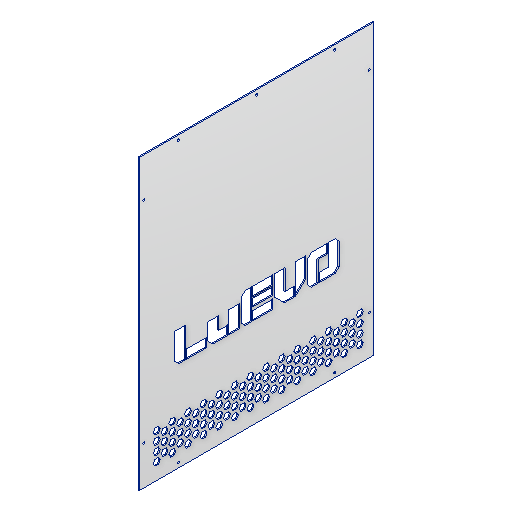
# Autodesk Inventor part: Camera Side Panel
Saved by Autodesk Inventor 2023.2 (Build 272271000, 271)
## iProperties
Created: 2023-02-06
Part Number: Camera Side Panel
Material: Aluminum 6061
Document SubType Name: Modeling
Designer: remop
Density: 2.7 g/cm^3
Appearance: Aluminum - Flat
Author: remop
Autodesk Inventor part; units mm, degrees
(part 1 of 2)
ref_plane "YZ Plane" through (0, 0, 0) normal (1, 0, 0) x (0, 1, 0)
ref_plane "XZ Plane" through (0, 0, 0) normal (0, 1, 0) x (-1, 0, 0)
ref_plane "XY Plane" through (0, 0, 0) normal (0, 0, 1) x (1, 0, 0)
sketch "Sketch1" plane through (0, 0, 0) normal (1, 0, 0) x (0, 1, 0)
  line L0 (168.0981, 15.8482) -> (163.0981, 18.735) projected
  line L1 (163.0981, 18.735) -> (163.0981, 24.5085) projected
  line L2 (163.0981, 24.5085) -> (168.0981, 27.3952) projected
  line L3 (168.0981, 27.3952) -> (173.0981, 24.5085) projected
  line L4 (173.0981, 24.5085) -> (173.0981, 18.735) projected
  line L5 (173.0981, 18.735) -> (168.0981, 15.8482) projected
  line L6 (130.5981, 40.3856) -> (135.5981, 37.4988) projected
  line L7 (135.5981, 37.4988) -> (135.5981, 31.7253) projected
  line L8 (135.5981, 31.7253) -> (130.5981, 28.8386) projected
  line L9 (130.5981, 28.8386) -> (125.5981, 31.7253) projected
  line L10 (125.5981, 31.7253) -> (125.5981, 37.4988) projected
  line L11 (125.5981, 37.4988) -> (130.5981, 40.3856) projected
  line L12 (158.0981, 50.5085) -> (158.0981, 44.735) projected
  line L13 (158.0981, 44.735) -> (153.0981, 41.8482) projected
  line L14 (153.0981, 41.8482) -> (148.0981, 44.735) projected
  line L15 (148.0981, 44.735) -> (148.0981, 50.5085) projected
  line L16 (148.0981, 50.5085) -> (153.0981, 53.3952) projected
  line L17 (153.0981, 53.3952) -> (158.0981, 50.5085) projected
  line L18 (140.5981, 63.4988) -> (145.5981, 66.3856) projected
  line L19 (145.5981, 66.3856) -> (150.5981, 63.4988) projected
  line L20 (150.5981, 63.4988) -> (150.5981, 57.7253) projected
  line L21 (150.5981, 57.7253) -> (145.5981, 54.8386) projected
  line L22 (145.5981, 54.8386) -> (140.5981, 57.7253) projected
  line L23 (140.5981, 57.7253) -> (140.5981, 63.4988) projected
  line L24 (143.0981, 70.735) -> (138.0981, 67.8482) projected
  line L25 (138.0981, 67.8482) -> (133.0981, 70.735) projected
  line L26 (133.0981, 70.735) -> (133.0981, 76.5085) projected
  line L27 (133.0981, 76.5085) -> (138.0981, 79.3952) projected
  line L28 (138.0981, 79.3952) -> (143.0981, 76.5085) projected
  line L29 (143.0981, 76.5085) -> (143.0981, 70.735) projected
  line L30 (160.5981, 92.3856) -> (165.5981, 89.4988) projected
  line L31 (165.5981, 89.4988) -> (165.5981, 83.7253) projected
  line L32 (165.5981, 83.7253) -> (160.5981, 80.8386) projected
  line L33 (160.5981, 80.8386) -> (155.5981, 83.7253) projected
  line L34 (155.5981, 83.7253) -> (155.5981, 89.4988) projected
  line L35 (155.5981, 89.4988) -> (160.5981, 92.3856) projected
  line L36 (128.0981, 102.5085) -> (128.0981, 96.735) projected
  line L37 (128.0981, 96.735) -> (123.0981, 93.8482) projected
  line L38 (123.0981, 93.8482) -> (118.0981, 96.735) projected
  line L39 (118.0981, 96.735) -> (118.0981, 102.5085) projected
  line L40 (118.0981, 102.5085) -> (123.0981, 105.3952) projected
  line L41 (123.0981, 105.3952) -> (128.0981, 102.5085) projected
  line L42 (168.0981, 119.8482) -> (163.0981, 122.735) projected
  line L43 (163.0981, 122.735) -> (163.0981, 128.5085) projected
  line L44 (163.0981, 128.5085) -> (168.0981, 131.3952) projected
  line L45 (168.0981, 131.3952) -> (173.0981, 128.5085) projected
  line L46 (173.0981, 128.5085) -> (173.0981, 122.735) projected
  line L47 (173.0981, 122.735) -> (168.0981, 119.8482) projected
  line L48 (130.5981, 144.3856) -> (135.5981, 141.4988) projected
  line L49 (135.5981, 141.4988) -> (135.5981, 135.7253) projected
  line L50 (135.5981, 135.7253) -> (130.5981, 132.8386) projected
  line L51 (130.5981, 132.8386) -> (125.5981, 135.7253) projected
  line L52 (125.5981, 135.7253) -> (125.5981, 141.4988) projected
  line L53 (125.5981, 141.4988) -> (130.5981, 144.3856) projected
  line L54 (160.5981, 144.3856) -> (165.5981, 141.4988) projected
  line L55 (165.5981, 141.4988) -> (165.5981, 135.7253) projected
  line L56 (165.5981, 135.7253) -> (160.5981, 132.8386) projected
  line L57 (160.5981, 132.8386) -> (155.5981, 135.7253) projected
  line L58 (155.5981, 135.7253) -> (155.5981, 141.4988) projected
  line L59 (155.5981, 141.4988) -> (160.5981, 144.3856) projected
  line L60 (140.5981, 167.4988) -> (145.5981, 170.3856) projected
  line L61 (145.5981, 170.3856) -> (150.5981, 167.4988) projected
  line L62 (150.5981, 167.4988) -> (150.5981, 161.7253) projected
  line L63 (150.5981, 161.7253) -> (145.5981, 158.8386) projected
  line L64 (145.5981, 158.8386) -> (140.5981, 161.7253) projected
  line L65 (140.5981, 161.7253) -> (140.5981, 167.4988) projected
  line L66 (143.0981, 174.735) -> (138.0981, 171.8482) projected
  line L67 (138.0981, 171.8482) -> (133.0981, 174.735) projected
  line L68 (133.0981, 174.735) -> (133.0981, 180.5085) projected
  line L69 (133.0981, 180.5085) -> (138.0981, 183.3952) projected
  line L70 (138.0981, 183.3952) -> (143.0981, 180.5085) projected
  line L71 (143.0981, 180.5085) -> (143.0981, 174.735) projected
  line L72 (160.5981, 196.3856) -> (165.5981, 193.4988) projected
  line L73 (165.5981, 193.4988) -> (165.5981, 187.7253) projected
  line L74 (165.5981, 187.7253) -> (160.5981, 184.8386) projected
  line L75 (160.5981, 184.8386) -> (155.5981, 187.7253) projected
  line L76 (155.5981, 187.7253) -> (155.5981, 193.4988) projected
  line L77 (155.5981, 193.4988) -> (160.5981, 196.3856) projected
  line L78 (128.0981, 206.5085) -> (128.0981, 200.735) projected
  line L79 (128.0981, 200.735) -> (123.0981, 197.8482) projected
  line L80 (123.0981, 197.8482) -> (118.0981, 200.735) projected
  line L81 (118.0981, 200.735) -> (118.0981, 206.5085) projected
  line L82 (118.0981, 206.5085) -> (123.0981, 209.3952) projected
  line L83 (123.0981, 209.3952) -> (128.0981, 206.5085) projected
  line L84 (168.0981, 223.8482) -> (163.0981, 226.735) projected
  line L85 (163.0981, 226.735) -> (163.0981, 232.5085) projected
  line L86 (163.0981, 232.5085) -> (168.0981, 235.3952) projected
  line L87 (168.0981, 235.3952) -> (173.0981, 232.5085) projected
  line L88 (173.0981, 232.5085) -> (173.0981, 226.735) projected
  line L89 (173.0981, 226.735) -> (168.0981, 223.8482) projected
  line L90 (130.5981, 248.3856) -> (135.5981, 245.4988) projected
  line L91 (135.5981, 245.4988) -> (135.5981, 239.7253) projected
  line L92 (135.5981, 239.7253) -> (130.5981, 236.8386) projected
  line L93 (130.5981, 236.8386) -> (125.5981, 239.7253) projected
  line L94 (125.5981, 239.7253) -> (125.5981, 245.4988) projected
  line L95 (125.5981, 245.4988) -> (130.5981, 248.3856) projected
  line L96 (158.0981, 258.5085) -> (158.0981, 252.735) projected
  line L97 (158.0981, 252.735) -> (153.0981, 249.8482) projected
  line L98 (153.0981, 249.8482) -> (148.0981, 252.735) projected
  line L99 (148.0981, 252.735) -> (148.0981, 258.5085) projected
  line L100 (148.0981, 258.5085) -> (153.0981, 261.3952) projected
  line L101 (153.0981, 261.3952) -> (158.0981, 258.5085) projected
  line L102 (128.0981, 284.5085) -> (128.0981, 278.735) projected
  line L103 (128.0981, 278.735) -> (123.0981, 275.8482) projected
  line L104 (123.0981, 275.8482) -> (118.0981, 278.735) projected
  line L105 (118.0981, 278.735) -> (118.0981, 284.5085) projected
  line L106 (118.0981, 284.5085) -> (123.0981, 287.3952) projected
  line L107 (123.0981, 287.3952) -> (128.0981, 284.5085) projected
  line L108 (128.0981, 336.5085) -> (128.0981, 330.735) projected
  line L109 (128.0981, 330.735) -> (123.0981, 327.8482) projected
  line L110 (123.0981, 327.8482) -> (118.0981, 330.735) projected
  line L111 (118.0981, 330.735) -> (118.0981, 336.5085) projected
  line L112 (118.0981, 336.5085) -> (123.0981, 339.3952) projected
  line L113 (123.0981, 339.3952) -> (128.0981, 336.5085) projected
  line L114 (160.5981, 326.3856) -> (165.5981, 323.4988) projected
  line L115 (165.5981, 323.4988) -> (165.5981, 317.7253) projected
  line L116 (165.5981, 317.7253) -> (160.5981, 314.8386) projected
  line L117 (160.5981, 314.8386) -> (155.5981, 317.7253) projected
  line L118 (155.5981, 317.7253) -> (155.5981, 323.4988) projected
  line L119 (155.5981, 323.4988) -> (160.5981, 326.3856) projected
  line L120 (140.5981, 271.4988) -> (145.5981, 274.3856) projected
  line L121 (145.5981, 274.3856) -> (150.5981, 271.4988) projected
  line L122 (150.5981, 271.4988) -> (150.5981, 265.7253) projected
  line L123 (150.5981, 265.7253) -> (145.5981, 262.8386) projected
  line L124 (145.5981, 262.8386) -> (140.5981, 265.7253) projected
  line L125 (140.5981, 265.7253) -> (140.5981, 271.4988) projected
  line L126 (160.5981, 300.3856) -> (165.5981, 297.4988) projected
  line L127 (165.5981, 297.4988) -> (165.5981, 291.7253) projected
  line L128 (165.5981, 291.7253) -> (160.5981, 288.8386) projected
  line L129 (160.5981, 288.8386) -> (155.5981, 291.7253) projected
  line L130 (155.5981, 291.7253) -> (155.5981, 297.4988) projected
  line L131 (155.5981, 297.4988) -> (160.5981, 300.3856) projected
  line L132 (143.0981, -1.4915) -> (143.0981, -7.265) projected
  line L133 (143.0981, -7.265) -> (138.0981, -10.1518) projected
  line L134 (138.0981, -10.1518) -> (133.0981, -7.265) projected
  line L135 (133.0981, -7.265) -> (133.0981, -1.4915) projected
  line L136 (133.0981, -1.4915) -> (138.0981, 1.3952) projected
  line L137 (138.0981, 1.3952) -> (143.0981, -1.4915) projected
  line L138 (130.5981, 14.3856) -> (135.5981, 11.4988) projected
  line L139 (135.5981, 11.4988) -> (135.5981, 5.7253) projected
  line L140 (135.5981, 5.7253) -> (130.5981, 2.8386) projected
  line L141 (130.5981, 2.8386) -> (125.5981, 5.7253) projected
  line L142 (125.5981, 5.7253) -> (125.5981, 11.4988) projected
  line L143 (125.5981, 11.4988) -> (130.5981, 14.3856) projected
  line L144 (148.0981, -7.265) -> (148.0981, -1.4915) projected
  line L145 (148.0981, -1.4915) -> (153.0981, 1.3952) projected
  line L146 (153.0981, 1.3952) -> (158.0981, -1.4915) projected
  line L147 (158.0981, -1.4915) -> (158.0981, -7.265) projected
  line L148 (158.0981, -7.265) -> (153.0981, -10.1518) projected
  line L149 (153.0981, -10.1518) -> (148.0981, -7.265) projected
  line L150 (158.0981, 310.5085) -> (158.0981, 304.735) projected
  line L151 (158.0981, 304.735) -> (153.0981, 301.8482) projected
  line L152 (153.0981, 301.8482) -> (148.0981, 304.735) projected
  line L153 (148.0981, 304.735) -> (148.0981, 310.5085) projected
  line L154 (148.0981, 310.5085) -> (153.0981, 313.3952) projected
  line L155 (153.0981, 313.3952) -> (158.0981, 310.5085) projected
  line L156 (158.0981, 284.5085) -> (158.0981, 278.735) projected
  line L157 (158.0981, 278.735) -> (153.0981, 275.8482) projected
  line L158 (153.0981, 275.8482) -> (148.0981, 278.735) projected
  line L159 (148.0981, 278.735) -> (148.0981, 284.5085) projected
  line L160 (148.0981, 284.5085) -> (153.0981, 287.3952) projected
  line L161 (153.0981, 287.3952) -> (158.0981, 284.5085) projected
  line L162 (168.0981, 301.8482) -> (163.0981, 304.735) projected
  line L163 (163.0981, 304.735) -> (163.0981, 310.5085) projected
  line L164 (163.0981, 310.5085) -> (168.0981, 313.3952) projected
  line L165 (168.0981, 313.3952) -> (173.0981, 310.5085) projected
  line L166 (173.0981, 310.5085) -> (173.0981, 304.735) projected
  line L167 (173.0981, 304.735) -> (168.0981, 301.8482) projected
  line L168 (143.0981, 330.735) -> (138.0981, 327.8482) projected
  line L169 (138.0981, 327.8482) -> (133.0981, 330.735) projected
  line L170 (133.0981, 330.735) -> (133.0981, 336.5085) projected
  line L171 (133.0981, 336.5085) -> (138.0981, 339.3952) projected
  line L172 (138.0981, 339.3952) -> (143.0981, 336.5085) projected
  line L173 (143.0981, 336.5085) -> (143.0981, 330.735) projected
  line L174 (130.5981, 300.3856) -> (135.5981, 297.4988) projected
  line L175 (135.5981, 297.4988) -> (135.5981, 291.7253) projected
  line L176 (135.5981, 291.7253) -> (130.5981, 288.8386) projected
  line L177 (130.5981, 288.8386) -> (125.5981, 291.7253) projected
  line L178 (125.5981, 291.7253) -> (125.5981, 297.4988) projected
  line L179 (125.5981, 297.4988) -> (130.5981, 300.3856) projected
  line L180 (143.0981, 252.735) -> (138.0981, 249.8482) projected
  line L181 (138.0981, 249.8482) -> (133.0981, 252.735) projected
  line L182 (133.0981, 252.735) -> (133.0981, 258.5085) projected
  line L183 (133.0981, 258.5085) -> (138.0981, 261.3952) projected
  line L184 (138.0981, 261.3952) -> (143.0981, 258.5085) projected
  line L185 (143.0981, 258.5085) -> (143.0981, 252.735) projected
  line L186 (140.5981, 245.4988) -> (145.5981, 248.3856) projected
  line L187 (145.5981, 248.3856) -> (150.5981, 245.4988) projected
  line L188 (150.5981, 245.4988) -> (150.5981, 239.7253) projected
  line L189 (150.5981, 239.7253) -> (145.5981, 236.8386) projected
  line L190 (145.5981, 236.8386) -> (140.5981, 239.7253) projected
  line L191 (140.5981, 239.7253) -> (140.5981, 245.4988) projected
  line L192 (158.0981, 232.5085) -> (158.0981, 226.735) projected
  line L193 (158.0981, 226.735) -> (153.0981, 223.8482) projected
  line L194 (153.0981, 223.8482) -> (148.0981, 226.735) projected
  line L195 (148.0981, 226.735) -> (148.0981, 232.5085) projected
  line L196 (148.0981, 232.5085) -> (153.0981, 235.3952) projected
  line L197 (153.0981, 235.3952) -> (158.0981, 232.5085) projected
  line L198 (130.5981, 222.3856) -> (135.5981, 219.4988) projected
  line L199 (135.5981, 219.4988) -> (135.5981, 213.7253) projected
  line L200 (135.5981, 213.7253) -> (130.5981, 210.8386) projected
  line L201 (130.5981, 210.8386) -> (125.5981, 213.7253) projected
  line L202 (125.5981, 213.7253) -> (125.5981, 219.4988) projected
  line L203 (125.5981, 219.4988) -> (130.5981, 222.3856) projected
  line L204 (168.0981, 197.8482) -> (163.0981, 200.735) projected
  line L205 (163.0981, 200.735) -> (163.0981, 206.5085) projected
  line L206 (163.0981, 206.5085) -> (168.0981, 209.3952) projected
  line L207 (168.0981, 209.3952) -> (173.0981, 206.5085) projected
  line L208 (173.0981, 206.5085) -> (173.0981, 200.735) projected
  line L209 (173.0981, 200.735) -> (168.0981, 197.8482) projected
  line L210 (128.0981, 180.5085) -> (128.0981, 174.735) projected
  line L211 (128.0981, 174.735) -> (123.0981, 171.8482) projected
  line L212 (123.0981, 171.8482) -> (118.0981, 174.735) projected
  line L213 (118.0981, 174.735) -> (118.0981, 180.5085) projected
  line L214 (118.0981, 180.5085) -> (123.0981, 183.3952) projected
  line L215 (123.0981, 183.3952) -> (128.0981, 180.5085) projected
  line L216 (160.5981, 170.3856) -> (165.5981, 167.4988) projected
  line L217 (165.5981, 167.4988) -> (165.5981, 161.7253) projected
  line L218 (165.5981, 161.7253) -> (160.5981, 158.8386) projected
  line L219 (160.5981, 158.8386) -> (155.5981, 161.7253) projected
  line L220 (155.5981, 161.7253) -> (155.5981, 167.4988) projected
  line L221 (155.5981, 167.4988) -> (160.5981, 170.3856) projected
  line L222 (168.0981, 145.8482) -> (163.0981, 148.735) projected
  line L223 (163.0981, 148.735) -> (163.0981, 154.5085) projected
  line L224 (163.0981, 154.5085) -> (168.0981, 157.3952) projected
  line L225 (168.0981, 157.3952) -> (173.0981, 154.5085) projected
  line L226 (173.0981, 154.5085) -> (173.0981, 148.735) projected
  line L227 (173.0981, 148.735) -> (168.0981, 145.8482) projected
  line L228 (128.0981, 154.5085) -> (128.0981, 148.735) projected
  line L229 (128.0981, 148.735) -> (123.0981, 145.8482) projected
  line L230 (123.0981, 145.8482) -> (118.0981, 148.735) projected
  line L231 (118.0981, 148.735) -> (118.0981, 154.5085) projected
  line L232 (118.0981, 154.5085) -> (123.0981, 157.3952) projected
  line L233 (123.0981, 157.3952) -> (128.0981, 154.5085) projected
  line L234 (158.0981, 128.5085) -> (158.0981, 122.735) projected
  line L235 (158.0981, 122.735) -> (153.0981, 119.8482) projected
  line L236 (153.0981, 119.8482) -> (148.0981, 122.735) projected
  line L237 (148.0981, 122.735) -> (148.0981, 128.5085) projected
  line L238 (148.0981, 128.5085) -> (153.0981, 131.3952) projected
  line L239 (153.0981, 131.3952) -> (158.0981, 128.5085) projected
  line L240 (130.5981, 118.3856) -> (135.5981, 115.4988) projected
  line L241 (135.5981, 115.4988) -> (135.5981, 109.7253) projected
  line L242 (135.5981, 109.7253) -> (130.5981, 106.8386) projected
  line L243 (130.5981, 106.8386) -> (125.5981, 109.7253) projected
  line L244 (125.5981, 109.7253) -> (125.5981, 115.4988) projected
  line L245 (125.5981, 115.4988) -> (130.5981, 118.3856) projected
  line L246 (168.0981, 93.8482) -> (163.0981, 96.735) projected
  line L247 (163.0981, 96.735) -> (163.0981, 102.5085) projected
  line L248 (163.0981, 102.5085) -> (168.0981, 105.3952) projected
  line L249 (168.0981, 105.3952) -> (173.0981, 102.5085) projected
  line L250 (173.0981, 102.5085) -> (173.0981, 96.735) projected
  line L251 (173.0981, 96.735) -> (168.0981, 93.8482) projected
  line L252 (128.0981, 76.5085) -> (128.0981, 70.735) projected
  line L253 (128.0981, 70.735) -> (123.0981, 67.8482) projected
  line L254 (123.0981, 67.8482) -> (118.0981, 70.735) projected
  line L255 (118.0981, 70.735) -> (118.0981, 76.5085) projected
  line L256 (118.0981, 76.5085) -> (123.0981, 79.3952) projected
  line L257 (123.0981, 79.3952) -> (128.0981, 76.5085) projected
  line L258 (160.5981, 66.3856) -> (165.5981, 63.4988) projected
  line L259 (165.5981, 63.4988) -> (165.5981, 57.7253) projected
  line L260 (165.5981, 57.7253) -> (160.5981, 54.8386) projected
  line L261 (160.5981, 54.8386) -> (155.5981, 57.7253) projected
  line L262 (155.5981, 57.7253) -> (155.5981, 63.4988) projected
  line L263 (155.5981, 63.4988) -> (160.5981, 66.3856) projected
  line L264 (143.0981, 44.735) -> (138.0981, 41.8482) projected
  line L265 (138.0981, 41.8482) -> (133.0981, 44.735) projected
  line L266 (133.0981, 44.735) -> (133.0981, 50.5085) projected
  line L267 (133.0981, 50.5085) -> (138.0981, 53.3952) projected
  line L268 (138.0981, 53.3952) -> (143.0981, 50.5085) projected
  line L269 (143.0981, 50.5085) -> (143.0981, 44.735) projected
  line L270 (140.5981, 37.4988) -> (145.5981, 40.3856) projected
  line L271 (145.5981, 40.3856) -> (150.5981, 37.4988) projected
  line L272 (150.5981, 37.4988) -> (150.5981, 31.7253) projected
  line L273 (150.5981, 31.7253) -> (145.5981, 28.8386) projected
  line L274 (145.5981, 28.8386) -> (140.5981, 31.7253) projected
  line L275 (140.5981, 31.7253) -> (140.5981, 37.4988) projected
  line L276 (158.0981, 24.5085) -> (158.0981, 18.735) projected
  line L277 (158.0981, 18.735) -> (153.0981, 15.8482) projected
  line L278 (153.0981, 15.8482) -> (148.0981, 18.735) projected
  line L279 (148.0981, 18.735) -> (148.0981, 24.5085) projected
  line L280 (148.0981, 24.5085) -> (153.0981, 27.3952) projected
  line L281 (153.0981, 27.3952) -> (158.0981, 24.5085) projected
  line L282 (155.5981, 5.7253) -> (155.5981, 11.4988) projected
  line L283 (155.5981, 11.4988) -> (160.5981, 14.3856) projected
  line L284 (160.5981, 14.3856) -> (165.5981, 11.4988) projected
  line L285 (165.5981, 11.4988) -> (165.5981, 5.7253) projected
  line L286 (165.5981, 5.7253) -> (160.5981, 2.8386) projected
  line L287 (160.5981, 2.8386) -> (155.5981, 5.7253) projected
  line L288 (128.0981, 24.5085) -> (128.0981, 18.735) projected
  line L289 (128.0981, 18.735) -> (123.0981, 15.8482) projected
  line L290 (123.0981, 15.8482) -> (118.0981, 18.735) projected
  line L291 (118.0981, 18.735) -> (118.0981, 24.5085) projected
  line L292 (118.0981, 24.5085) -> (123.0981, 27.3952) projected
  line L293 (123.0981, 27.3952) -> (128.0981, 24.5085) projected
  line L294 (168.0981, 41.8482) -> (163.0981, 44.735) projected
  line L295 (163.0981, 44.735) -> (163.0981, 50.5085) projected
  line L296 (163.0981, 50.5085) -> (168.0981, 53.3952) projected
  line L297 (168.0981, 53.3952) -> (173.0981, 50.5085) projected
  line L298 (173.0981, 50.5085) -> (173.0981, 44.735) projected
  line L299 (173.0981, 44.735) -> (168.0981, 41.8482) projected
  line L300 (130.5981, 66.3856) -> (135.5981, 63.4988) projected
  line L301 (135.5981, 63.4988) -> (135.5981, 57.7253) projected
  line L302 (135.5981, 57.7253) -> (130.5981, 54.8386) projected
  line L303 (130.5981, 54.8386) -> (125.5981, 57.7253) projected
  line L304 (125.5981, 57.7253) -> (125.5981, 63.4988) projected
  line L305 (125.5981, 63.4988) -> (130.5981, 66.3856) projected
  line L306 (158.0981, 76.5085) -> (158.0981, 70.735) projected
  line L307 (158.0981, 70.735) -> (153.0981, 67.8482) projected
  line L308 (153.0981, 67.8482) -> (148.0981, 70.735) projected
  line L309 (148.0981, 70.735) -> (148.0981, 76.5085) projected
  line L310 (148.0981, 76.5085) -> (153.0981, 79.3952) projected
  line L311 (153.0981, 79.3952) -> (158.0981, 76.5085) projected
  line L312 (140.5981, 89.4988) -> (145.5981, 92.3856) projected
  line L313 (145.5981, 92.3856) -> (150.5981, 89.4988) projected
  line L314 (150.5981, 89.4988) -> (150.5981, 83.7253) projected
  line L315 (150.5981, 83.7253) -> (145.5981, 80.8386) projected
  line L316 (145.5981, 80.8386) -> (140.5981, 83.7253) projected
  line L317 (140.5981, 83.7253) -> (140.5981, 89.4988) projected
  line L318 (143.0981, 96.735) -> (138.0981, 93.8482) projected
  line L319 (138.0981, 93.8482) -> (133.0981, 96.735) projected
  line L320 (133.0981, 96.735) -> (133.0981, 102.5085) projected
  line L321 (133.0981, 102.5085) -> (138.0981, 105.3952) projected
  line L322 (138.0981, 105.3952) -> (143.0981, 102.5085) projected
  line L323 (143.0981, 102.5085) -> (143.0981, 96.735) projected
  line L324 (160.5981, 118.3856) -> (165.5981, 115.4988) projected
  line L325 (165.5981, 115.4988) -> (165.5981, 109.7253) projected
  line L326 (165.5981, 109.7253) -> (160.5981, 106.8386) projected
  line L327 (160.5981, 106.8386) -> (155.5981, 109.7253) projected
  line L328 (155.5981, 109.7253) -> (155.5981, 115.4988) projected
  line L329 (155.5981, 115.4988) -> (160.5981, 118.3856) projected
  line L330 (128.0981, 128.5085) -> (128.0981, 122.735) projected
  line L331 (128.0981, 122.735) -> (123.0981, 119.8482) projected
  line L332 (123.0981, 119.8482) -> (118.0981, 122.735) projected
  line L333 (118.0981, 122.735) -> (118.0981, 128.5085) projected
  line L334 (118.0981, 128.5085) -> (123.0981, 131.3952) projected
  line L335 (123.0981, 131.3952) -> (128.0981, 128.5085) projected
  line L336 (140.5981, 141.4988) -> (145.5981, 144.3856) projected
  line L337 (145.5981, 144.3856) -> (150.5981, 141.4988) projected
  line L338 (150.5981, 141.4988) -> (150.5981, 135.7253) projected
  line L339 (150.5981, 135.7253) -> (145.5981, 132.8386) projected
  line L340 (145.5981, 132.8386) -> (140.5981, 135.7253) projected
  line L341 (140.5981, 135.7253) -> (140.5981, 141.4988) projected
  line L342 (130.5981, 170.3856) -> (135.5981, 167.4988) projected
  line L343 (135.5981, 167.4988) -> (135.5981, 161.7253) projected
  line L344 (135.5981, 161.7253) -> (130.5981, 158.8386) projected
  line L345 (130.5981, 158.8386) -> (125.5981, 161.7253) projected
  line L346 (125.5981, 161.7253) -> (125.5981, 167.4988) projected
  line L347 (125.5981, 167.4988) -> (130.5981, 170.3856) projected
  line L348 (158.0981, 180.5085) -> (158.0981, 174.735) projected
  line L349 (158.0981, 174.735) -> (153.0981, 171.8482) projected
  line L350 (153.0981, 171.8482) -> (148.0981, 174.735) projected
  line L351 (148.0981, 174.735) -> (148.0981, 180.5085) projected
  line L352 (148.0981, 180.5085) -> (153.0981, 183.3952) projected
  line L353 (153.0981, 183.3952) -> (158.0981, 180.5085) projected
  line L354 (140.5981, 193.4988) -> (145.5981, 196.3856) projected
  line L355 (145.5981, 196.3856) -> (150.5981, 193.4988) projected
  line L356 (150.5981, 193.4988) -> (150.5981, 187.7253) projected
  line L357 (150.5981, 187.7253) -> (145.5981, 184.8386) projected
  line L358 (145.5981, 184.8386) -> (140.5981, 187.7253) projected
  line L359 (140.5981, 187.7253) -> (140.5981, 193.4988) projected
  line L360 (143.0981, 200.735) -> (138.0981, 197.8482) projected
  line L361 (138.0981, 197.8482) -> (133.0981, 200.735) projected
  line L362 (133.0981, 200.735) -> (133.0981, 206.5085) projected
  line L363 (133.0981, 206.5085) -> (138.0981, 209.3952) projected
  line L364 (138.0981, 209.3952) -> (143.0981, 206.5085) projected
  line L365 (143.0981, 206.5085) -> (143.0981, 200.735) projected
  line L366 (160.5981, 222.3856) -> (165.5981, 219.4988) projected
  line L367 (165.5981, 219.4988) -> (165.5981, 213.7253) projected
  line L368 (165.5981, 213.7253) -> (160.5981, 210.8386) projected
  line L369 (160.5981, 210.8386) -> (155.5981, 213.7253) projected
  line L370 (155.5981, 213.7253) -> (155.5981, 219.4988) projected
  line L371 (155.5981, 219.4988) -> (160.5981, 222.3856) projected
  line L372 (128.0981, 232.5085) -> (128.0981, 226.735) projected
  line L373 (128.0981, 226.735) -> (123.0981, 223.8482) projected
  line L374 (123.0981, 223.8482) -> (118.0981, 226.735) projected
  line L375 (118.0981, 226.735) -> (118.0981, 232.5085) projected
  line L376 (118.0981, 232.5085) -> (123.0981, 235.3952) projected
  line L377 (123.0981, 235.3952) -> (128.0981, 232.5085) projected
  line L378 (168.0981, 249.8482) -> (163.0981, 252.735) projected
  line L379 (163.0981, 252.735) -> (163.0981, 258.5085) projected
  line L380 (163.0981, 258.5085) -> (168.0981, 261.3952) projected
  line L381 (168.0981, 261.3952) -> (173.0981, 258.5085) projected
  line L382 (173.0981, 258.5085) -> (173.0981, 252.735) projected
  line L383 (173.0981, 252.735) -> (168.0981, 249.8482) projected
  line L384 (130.5981, 274.3856) -> (135.5981, 271.4988) projected
  line L385 (135.5981, 271.4988) -> (135.5981, 265.7253) projected
  line L386 (135.5981, 265.7253) -> (130.5981, 262.8386) projected
  line L387 (130.5981, 262.8386) -> (125.5981, 265.7253) projected
  line L388 (125.5981, 265.7253) -> (125.5981, 271.4988) projected
  line L389 (125.5981, 271.4988) -> (130.5981, 274.3856) projected
  line L390 (130.5981, 326.3856) -> (135.5981, 323.4988) projected
  line L391 (135.5981, 323.4988) -> (135.5981, 317.7253) projected
  line L392 (135.5981, 317.7253) -> (130.5981, 314.8386) projected
  line L393 (130.5981, 314.8386) -> (125.5981, 317.7253) projected
  line L394 (125.5981, 317.7253) -> (125.5981, 323.4988) projected
  line L395 (125.5981, 323.4988) -> (130.5981, 326.3856) projected
  line L396 (168.0981, 327.8482) -> (163.0981, 330.735) projected
  line L397 (163.0981, 330.735) -> (163.0981, 336.5085) projected
  line L398 (163.0981, 336.5085) -> (168.0981, 339.3952) projected
  line L399 (168.0981, 339.3952) -> (173.0981, 336.5085) projected
  line L400 (173.0981, 336.5085) -> (173.0981, 330.735) projected
  line L401 (173.0981, 330.735) -> (168.0981, 327.8482) projected
  line L402 (160.5981, 274.3856) -> (165.5981, 271.4988) projected
  line L403 (165.5981, 271.4988) -> (165.5981, 265.7253) projected
  line L404 (165.5981, 265.7253) -> (160.5981, 262.8386) projected
  line L405 (160.5981, 262.8386) -> (155.5981, 265.7253) projected
  line L406 (155.5981, 265.7253) -> (155.5981, 271.4988) projected
  line L407 (155.5981, 271.4988) -> (160.5981, 274.3856) projected
  line L408 (140.5981, 297.4988) -> (145.5981, 300.3856) projected
  line L409 (145.5981, 300.3856) -> (150.5981, 297.4988) projected
  line L410 (150.5981, 297.4988) -> (150.5981, 291.7253) projected
  line L411 (150.5981, 291.7253) -> (145.5981, 288.8386) projected
  line L412 (145.5981, 288.8386) -> (140.5981, 291.7253) projected
  line L413 (140.5981, 291.7253) -> (140.5981, 297.4988) projected
  line L414 (140.5981, 323.4988) -> (145.5981, 326.3856) projected
  line L415 (145.5981, 326.3856) -> (150.5981, 323.4988) projected
  line L416 (150.5981, 323.4988) -> (150.5981, 317.7253) projected
  line L417 (150.5981, 317.7253) -> (145.5981, 314.8386) projected
  line L418 (145.5981, 314.8386) -> (140.5981, 317.7253) projected
  line L419 (140.5981, 317.7253) -> (140.5981, 323.4988) projected
  line L420 (140.5981, 5.7253) -> (140.5981, 11.4988) projected
  line L421 (140.5981, 11.4988) -> (145.5981, 14.3856) projected
  line L422 (145.5981, 14.3856) -> (150.5981, 11.4988) projected
  line L423 (150.5981, 11.4988) -> (150.5981, 5.7253) projected
  line L424 (150.5981, 5.7253) -> (145.5981, 2.8386) projected
  line L425 (145.5981, 2.8386) -> (140.5981, 5.7253) projected
  line L426 (128.0981, -1.4915) -> (128.0981, -7.265) projected
  line L427 (128.0981, -7.265) -> (123.0981, -10.1518) projected
  line L428 (123.0981, -10.1518) -> (118.0981, -7.265) projected
  line L429 (118.0981, -7.265) -> (118.0981, -1.4915) projected
  line L430 (118.0981, -1.4915) -> (123.0981, 1.3952) projected
  line L431 (123.0981, 1.3952) -> (128.0981, -1.4915) projected
  line L432 (143.0981, 304.735) -> (138.0981, 301.8482) projected
  line L433 (138.0981, 301.8482) -> (133.0981, 304.735) projected
  line L434 (133.0981, 304.735) -> (133.0981, 310.5085) projected
  line L435 (133.0981, 310.5085) -> (138.0981, 313.3952) projected
  line L436 (138.0981, 313.3952) -> (143.0981, 310.5085) projected
  line L437 (143.0981, 310.5085) -> (143.0981, 304.735) projected
  line L438 (143.0981, 278.735) -> (138.0981, 275.8482) projected
  line L439 (138.0981, 275.8482) -> (133.0981, 278.735) projected
  line L440 (133.0981, 278.735) -> (133.0981, 284.5085) projected
  line L441 (133.0981, 284.5085) -> (138.0981, 287.3952) projected
  line L442 (138.0981, 287.3952) -> (143.0981, 284.5085) projected
  line L443 (143.0981, 284.5085) -> (143.0981, 278.735) projected
  line L444 (168.0981, 275.8482) -> (163.0981, 278.735) projected
  line L445 (163.0981, 278.735) -> (163.0981, 284.5085) projected
  line L446 (163.0981, 284.5085) -> (168.0981, 287.3952) projected
  line L447 (168.0981, 287.3952) -> (173.0981, 284.5085) projected
  line L448 (173.0981, 284.5085) -> (173.0981, 278.735) projected
  line L449 (173.0981, 278.735) -> (168.0981, 275.8482) projected
  line L450 (158.0981, 336.5085) -> (158.0981, 330.735) projected
  line L451 (158.0981, 330.735) -> (153.0981, 327.8482) projected
  line L452 (153.0981, 327.8482) -> (148.0981, 330.735) projected
  line L453 (148.0981, 330.735) -> (148.0981, 336.5085) projected
  line L454 (148.0981, 336.5085) -> (153.0981, 339.3952) projected
  line L455 (153.0981, 339.3952) -> (158.0981, 336.5085) projected
  line L456 (128.0981, 310.5085) -> (128.0981, 304.735) projected
  line L457 (128.0981, 304.735) -> (123.0981, 301.8482) projected
  line L458 (123.0981, 301.8482) -> (118.0981, 304.735) projected
  line L459 (118.0981, 304.735) -> (118.0981, 310.5085) projected
  line L460 (118.0981, 310.5085) -> (123.0981, 313.3952) projected
  line L461 (123.0981, 313.3952) -> (128.0981, 310.5085) projected
  line L462 (128.0981, 258.5085) -> (128.0981, 252.735) projected
  line L463 (128.0981, 252.735) -> (123.0981, 249.8482) projected
  line L464 (123.0981, 249.8482) -> (118.0981, 252.735) projected
  line L465 (118.0981, 252.735) -> (118.0981, 258.5085) projected
  line L466 (118.0981, 258.5085) -> (123.0981, 261.3952) projected
  line L467 (123.0981, 261.3952) -> (128.0981, 258.5085) projected
  line L468 (160.5981, 248.3856) -> (165.5981, 245.4988) projected
  line L469 (165.5981, 245.4988) -> (165.5981, 239.7253) projected
  line L470 (165.5981, 239.7253) -> (160.5981, 236.8386) projected
  line L471 (160.5981, 236.8386) -> (155.5981, 239.7253) projected
  line L472 (155.5981, 239.7253) -> (155.5981, 245.4988) projected
  line L473 (155.5981, 245.4988) -> (160.5981, 248.3856) projected
  line L474 (143.0981, 226.735) -> (138.0981, 223.8482) projected
  line L475 (138.0981, 223.8482) -> (133.0981, 226.735) projected
  line L476 (133.0981, 226.735) -> (133.0981, 232.5085) projected
  line L477 (133.0981, 232.5085) -> (138.0981, 235.3952) projected
  line L478 (138.0981, 235.3952) -> (143.0981, 232.5085) projected
  line L479 (143.0981, 232.5085) -> (143.0981, 226.735) projected
  line L480 (140.5981, 219.4988) -> (145.5981, 222.3856) projected
  line L481 (145.5981, 222.3856) -> (150.5981, 219.4988) projected
  line L482 (150.5981, 219.4988) -> (150.5981, 213.7253) projected
  line L483 (150.5981, 213.7253) -> (145.5981, 210.8386) projected
  line L484 (145.5981, 210.8386) -> (140.5981, 213.7253) projected
  line L485 (140.5981, 213.7253) -> (140.5981, 219.4988) projected
  line L486 (158.0981, 206.5085) -> (158.0981, 200.735) projected
  line L487 (158.0981, 200.735) -> (153.0981, 197.8482) projected
  line L488 (153.0981, 197.8482) -> (148.0981, 200.735) projected
  line L489 (148.0981, 200.735) -> (148.0981, 206.5085) projected
  line L490 (148.0981, 206.5085) -> (153.0981, 209.3952) projected
  line L491 (153.0981, 209.3952) -> (158.0981, 206.5085) projected
  line L492 (130.5981, 196.3856) -> (135.5981, 193.4988) projected
  line L493 (135.5981, 193.4988) -> (135.5981, 187.7253) projected
  line L494 (135.5981, 187.7253) -> (130.5981, 184.8386) projected
  line L495 (130.5981, 184.8386) -> (125.5981, 187.7253) projected
  line L496 (125.5981, 187.7253) -> (125.5981, 193.4988) projected
  line L497 (125.5981, 193.4988) -> (130.5981, 196.3856) projected
  line L498 (168.0981, 171.8482) -> (163.0981, 174.735) projected
  line L499 (163.0981, 174.735) -> (163.0981, 180.5085) projected
  line L500 (163.0981, 180.5085) -> (168.0981, 183.3952) projected
  line L501 (168.0981, 183.3952) -> (173.0981, 180.5085) projected
  line L502 (173.0981, 180.5085) -> (173.0981, 174.735) projected
  line L503 (173.0981, 174.735) -> (168.0981, 171.8482) projected
  line L504 (158.0981, 154.5085) -> (158.0981, 148.735) projected
  line L505 (158.0981, 148.735) -> (153.0981, 145.8482) projected
  line L506 (153.0981, 145.8482) -> (148.0981, 148.735) projected
  line L507 (148.0981, 148.735) -> (148.0981, 154.5085) projected
  line L508 (148.0981, 154.5085) -> (153.0981, 157.3952) projected
  line L509 (153.0981, 157.3952) -> (158.0981, 154.5085) projected
  line L510 (143.0981, 148.735) -> (138.0981, 145.8482) projected
  line L511 (138.0981, 145.8482) -> (133.0981, 148.735) projected
  line L512 (133.0981, 148.735) -> (133.0981, 154.5085) projected
  line L513 (133.0981, 154.5085) -> (138.0981, 157.3952) projected
  line L514 (138.0981, 157.3952) -> (143.0981, 154.5085) projected
  line L515 (143.0981, 154.5085) -> (143.0981, 148.735) projected
  line L516 (143.0981, 122.735) -> (138.0981, 119.8482) projected
  line L517 (138.0981, 119.8482) -> (133.0981, 122.735) projected
  line L518 (133.0981, 122.735) -> (133.0981, 128.5085) projected
  line L519 (133.0981, 128.5085) -> (138.0981, 131.3952) projected
  line L520 (138.0981, 131.3952) -> (143.0981, 128.5085) projected
  line L521 (143.0981, 128.5085) -> (143.0981, 122.735) projected
  line L522 (140.5981, 115.4988) -> (145.5981, 118.3856) projected
  line L523 (145.5981, 118.3856) -> (150.5981, 115.4988) projected
  line L524 (150.5981, 115.4988) -> (150.5981, 109.7253) projected
  line L525 (150.5981, 109.7253) -> (145.5981, 106.8386) projected
  line L526 (145.5981, 106.8386) -> (140.5981, 109.7253) projected
  line L527 (140.5981, 109.7253) -> (140.5981, 115.4988) projected
  line L528 (158.0981, 102.5085) -> (158.0981, 96.735) projected
  line L529 (158.0981, 96.735) -> (153.0981, 93.8482) projected
  line L530 (153.0981, 93.8482) -> (148.0981, 96.735) projected
  line L531 (148.0981, 96.735) -> (148.0981, 102.5085) projected
  line L532 (148.0981, 102.5085) -> (153.0981, 105.3952) projected
  line L533 (153.0981, 105.3952) -> (158.0981, 102.5085) projected
  line L534 (130.5981, 92.3856) -> (135.5981, 89.4988) projected
  line L535 (135.5981, 89.4988) -> (135.5981, 83.7253) projected
  line L536 (135.5981, 83.7253) -> (130.5981, 80.8386) projected
  line L537 (130.5981, 80.8386) -> (125.5981, 83.7253) projected
  line L538 (125.5981, 83.7253) -> (125.5981, 89.4988) projected
  line L539 (125.5981, 89.4988) -> (130.5981, 92.3856) projected
  line L540 (168.0981, 67.8482) -> (163.0981, 70.735) projected
  line L541 (163.0981, 70.735) -> (163.0981, 76.5085) projected
  line L542 (163.0981, 76.5085) -> (168.0981, 79.3952) projected
  line L543 (168.0981, 79.3952) -> (173.0981, 76.5085) projected
  line L544 (173.0981, 76.5085) -> (173.0981, 70.735) projected
  line L545 (173.0981, 70.735) -> (168.0981, 67.8482) projected
  line L546 (128.0981, 50.5085) -> (128.0981, 44.735) projected
  line L547 (128.0981, 44.735) -> (123.0981, 41.8482) projected
  line L548 (123.0981, 41.8482) -> (118.0981, 44.735) projected
  line L549 (118.0981, 44.735) -> (118.0981, 50.5085) projected
  line L550 (118.0981, 50.5085) -> (123.0981, 53.3952) projected
  line L551 (123.0981, 53.3952) -> (128.0981, 50.5085) projected
  line L552 (160.5981, 40.3856) -> (165.5981, 37.4988) projected
  line L553 (165.5981, 37.4988) -> (165.5981, 31.7253) projected
  line L554 (165.5981, 31.7253) -> (160.5981, 28.8386) projected
  line L555 (160.5981, 28.8386) -> (155.5981, 31.7253) projected
  line L556 (155.5981, 31.7253) -> (155.5981, 37.4988) projected
  line L557 (155.5981, 37.4988) -> (160.5981, 40.3856) projected
  line L558 (143.0981, 18.735) -> (138.0981, 15.8482) projected
  line L559 (138.0981, 15.8482) -> (133.0981, 18.735) projected
  line L560 (133.0981, 18.735) -> (133.0981, 24.5085) projected
  line L561 (133.0981, 24.5085) -> (138.0981, 27.3952) projected
  line L562 (138.0981, 27.3952) -> (143.0981, 24.5085) projected
  line L563 (143.0981, 24.5085) -> (143.0981, 18.735) projected
  line L564 (163.0981, -7.265) -> (163.0981, -1.4915) projected
  line L565 (163.0981, -1.4915) -> (168.0981, 1.3952) projected
  line L566 (168.0981, 1.3952) -> (173.0981, -1.4915) projected
  line L567 (173.0981, -1.4915) -> (173.0981, -7.265) projected
  line L568 (173.0981, -7.265) -> (168.0981, -10.1518) projected
  line L569 (168.0981, -10.1518) -> (163.0981, -7.265) projected
  circle A0 centre (470.5981, 255.5102) radius 15 projected
  circle A1 centre (470.5981, 167.5102) radius 15 projected
  circle A2 centre (470.5981, 79.5102) radius 15 projected
  circle A3 centre (455.0981, 64.0102) radius 1.75 projected
  circle A4 centre (486.0981, 95.0102) radius 1.75 projected
  circle A5 centre (455.0981, 152.0102) radius 1.75 projected
  circle A6 centre (486.0981, 183.0102) radius 1.75 projected
  circle A7 centre (455.0981, 271.0102) radius 1.75 projected
  circle A8 centre (486.0981, 271.0102) radius 1.75 projected
  circle A9 centre (486.0981, 240.0102) radius 1.75 projected
  circle A10 centre (455.0981, 240.0102) radius 1.75 projected
  circle A11 centre (486.0981, 152.0102) radius 1.75 projected
  circle A12 centre (455.0981, 183.0102) radius 1.75 projected
  circle A13 centre (486.0981, 64.0102) radius 1.75 projected
  circle A14 centre (455.0981, 95.0102) radius 1.75 projected
  line L570 (96.0981, 362.5102) -> (576.0981, 362.5102) projected
  line L571 (96.0981, -27.4898) -> (96.0981, 362.5102) projected
  line L572 (576.0981, -27.4898) -> (96.0981, -27.4898) projected
  line L573 (576.0981, 362.5102) -> (576.0981, -27.4898) projected
  circle A15 centre (551.0981, 87.5102) radius 1.75 projected
  circle A16 centre (568.5981, 167.5102) radius 1.75 projected
  circle A17 centre (511.0981, -19.9898) radius 1.75 projected
  circle A18 centre (161.0981, -19.9898) radius 1.75 projected
  circle A19 centre (511.0981, 355.0102) radius 1.75 projected
  circle A20 centre (161.0981, 355.0102) radius 1.75 projected
  circle A21 centre (568.5981, 37.5102) radius 1.75 projected
  circle A22 centre (568.5981, 297.5102) radius 1.75 projected
  circle A23 centre (103.5981, 297.5102) radius 1.75 projected
  circle A24 centre (103.5981, 37.5102) radius 1.75 projected
  circle A25 centre (551.0981, 167.5102) radius 1.75 projected
  circle A26 centre (551.0981, 247.5102) radius 1.75 projected
  line L574 (246.1213, 271.2974) -> (281.6696, 271.2974) projected
  line L575 (281.6696, 271.2974) -> (281.6696, 287.0502) projected
  line L576 (281.6696, 287.0502) -> (296.1213, 287.0502) projected
  line L577 (296.1213, 287.0502) -> (296.1213, 260.9349) projected
  line L578 (296.1213, 260.9349) -> (289.8481, 254.6152) projected
  line L579 (289.8481, 254.6152) -> (252.3945, 254.6152) projected
  line L580 (252.3945, 254.6152) -> (246.1213, 260.9349) projected
  line L581 (246.1213, 260.9349) -> (246.1213, 271.2974) projected
  line L582 (246.0748, 230.4981) -> (260.8982, 230.4981) projected
  line L583 (260.8982, 230.4981) -> (260.8982, 214.7453) projected
  line L584 (260.8982, 214.7453) -> (296.1213, 214.7453) projected
  line L585 (296.1213, 214.7453) -> (296.1213, 198.0632) projected
  line L586 (296.1213, 198.0632) -> (262.757, 198.0632) projected
  line L587 (262.757, 198.0632) -> (246.0748, 214.7453) projected
  line L588 (246.0748, 214.7453) -> (246.0748, 230.4981) projected
  line L589 (246.1213, 193.7881) -> (259.9224, 193.7881) projected
  line L590 (259.9224, 193.7881) -> (259.9224, 161.3532) projected
  line L591 (259.9224, 161.3532) -> (246.1213, 161.3532) projected
  line L592 (246.1213, 161.3532) -> (246.1213, 193.7881) projected
  line L593 (246.1213, 157.8216) -> (296.1213, 157.8216) projected
  line L594 (296.1213, 157.8216) -> (296.1213, 147.5056) projected
  line L595 (296.1213, 147.5056) -> (289.8481, 141.2323) projected
  line L596 (289.8481, 141.2323) -> (252.3945, 141.2323) projected
  line L597 (252.3945, 141.2323) -> (246.1213, 147.5056) projected
  line L598 (246.1213, 147.5056) -> (246.1213, 157.8216) projected
  line L599 (246.1678, 116.8364) -> (259.9689, 116.8364) projected
  line L600 (259.9689, 116.8364) -> (259.9689, 101.0836) projected
  line L601 (259.9689, 101.0836) -> (281.809, 101.0836) projected
  line L602 (281.809, 101.0836) -> (281.809, 84.4015) projected
  line L603 (281.809, 84.4015) -> (254.0209, 84.4015) projected
  line L604 (254.0209, 84.4015) -> (246.1678, 92.2546) projected
  line L605 (246.1678, 92.2546) -> (246.1678, 116.8364) projected
  line L606 (246.1213, 34.1227) -> (246.1213, 44.2992) projected
  line L607 (246.1213, 44.2992) -> (296.1213, 44.2992) projected
  line L608 (296.1213, 44.2992) -> (296.1213, 27.8494) projected
  line L609 (296.1213, 27.8494) -> (252.3945, 27.8494) projected
  line L610 (252.3945, 27.8494) -> (246.1213, 34.1227) projected
  line L611 (246.1213, 47.8308) -> (246.1213, 80.0799) projected
  line L612 (246.1213, 80.0799) -> (259.9224, 80.0799) projected
  line L613 (259.9224, 80.0799) -> (259.9224, 47.8308) projected
  line L614 (259.9224, 47.8308) -> (246.1213, 47.8308) projected
  line L615 (246.1678, 136.9572) -> (281.809, 136.9572) projected
  line L616 (281.809, 136.9572) -> (281.809, 120.2751) projected
  line L617 (281.809, 120.2751) -> (246.1678, 120.2751) projected
  line L618 (246.1678, 120.2751) -> (246.1678, 136.9572) projected
  line L619 (281.6696, 193.7881) -> (296.1213, 193.7881) projected
  line L620 (296.1213, 193.7881) -> (296.1213, 161.3532) projected
  line L621 (296.1213, 161.3532) -> (281.6696, 161.3532) projected
  line L622 (281.6696, 161.3532) -> (281.6696, 193.7881) projected
  line L623 (267.125, 193.7881) -> (278.138, 193.7881) projected
  line L624 (278.138, 193.7881) -> (278.138, 161.3532) projected
  line L625 (278.138, 161.3532) -> (267.125, 161.3532) projected
  line L626 (267.125, 161.3532) -> (267.125, 193.7881) projected
  line L627 (246.1213, 233.9368) -> (262.757, 250.3401) projected
  line L628 (262.757, 250.3401) -> (296.1213, 250.3401) projected
  line L629 (296.1213, 250.3401) -> (296.1213, 233.9368) projected
  line L630 (296.1213, 233.9368) -> (246.1213, 233.9368) projected
  line L631 (252.3945, 307.171) -> (289.8481, 307.171) projected
  line L632 (289.8481, 307.171) -> (296.1213, 300.8513) projected
  line L633 (296.1213, 300.8513) -> (296.1213, 290.4888) projected
  line L634 (296.1213, 290.4888) -> (259.9224, 290.4888) projected
  line L635 (259.9224, 290.4888) -> (259.9224, 274.6896) projected
  line L636 (259.9224, 274.6896) -> (246.1213, 274.6896) projected
  line L637 (246.1213, 274.6896) -> (246.1213, 300.8513) projected
  line L638 (246.1213, 300.8513) -> (252.3945, 307.171) projected
  point P0 (0, 0)
extrude "Extrusion1" add sketch "Sketch1" along normal blind 2 contours A0 | A1 | A2 | A3 | A4 | A5 | A6 | A7 | A8 | A9 | A10 | A11 | A12 | A13 | A14 | L570 L573 L572 L571 | A15 | A25 | A26 | L574 L575 L576 L577 L578 L579 L580 L581 | L582 L583 L584 L585 L586 L587 L588 | L589 L590 L591 L592 | L593 L594 L595 L596 L597 L598 | L599 L600 L601 L602 L603 L604 L605 | L606 L607 L608 L609 L610 | L611 L612 L613 L614 | L615 L616 L617 L618 | L619 L620 L621 L622 | L623 L624 L625 L626 | L627 L628 L629 L630 | L631 L632 L633 L634 L635 L636 L637 L638